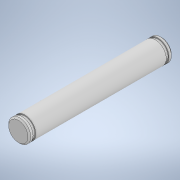
# Autodesk Inventor part: Aksel_stempel_bund
Saved by Autodesk Inventor 2022 (Build 260153000, 153)
## iProperties
Created: 2022-05-05
Part Number: Aksel_stempel_bund
Material: Generic
Document SubType Name: Modeling
Designer: patri
Density: 1 g/cm^3
Appearance: Default
Author: patri
Autodesk Inventor part; units mm, degrees
ref_plane "YZ Plane" through (0, 0, 0) normal (1, 0, 0) x (0, 1, 0)
ref_plane "XZ Plane" through (0, 0, 0) normal (0, 1, 0) x (-1, 0, 0)
ref_plane "XY Plane" through (0, 0, 0) normal (0, 0, 1) x (1, 0, 0)
sketch "Sketch1" plane through (0, 0, 0) normal (0, 1, 0) x (-1, 0, 0)
  line L0 (0, 0) -> (6, 0)
  line L1 (6, 0) -> (6, -78)
  line L2 (6, -78) -> (0, -78)
  line L3 (0, -78) -> (0, 0)
  line L4 (6, -2) -> (5.5, -2)
  line L5 (5.5, -2) -> (5.5, -3.5)
  line L6 (5.5, -3.5) -> (6, -3.5)
  line L7 (6, -3.5) -> (6, -2)
  line L8 (6, -76) -> (5.5, -76)
  line L9 (5.5, -76) -> (5.5, -74.5)
  line L10 (5.5, -74.5) -> (6, -74.5)
  line L11 (6, -74.5) -> (6, -76)
  point P0 (6, -74.5)
  point P1 (6, -3.5)
  dimension "d0" = 6
  dimension "d3" = 71
  dimension "d4" = 1.5
  dimension "d5" = 0.5
  dimension "d6" = 1.5
  dimension "d7" = 2
  dimension "d8" = 2
  constraints: 24 end point, 6 parallel, 3 horizontal, 3 perpendicular, 3 point on line
  measures "d0" distance between parallel lines of L3 L1
  measures "d3" distance between parallel lines of L6 L10
  measures "d4" distance of L4.end L5.end
  measures "d5" distance of L5.end L6.end
  measures "d6" distance of L8.end L9.end
  measures "d7" distance between parallel lines of L8 L2
  measures "d8" distance between parallel lines of L0 L4
revolve "Revolution1" add sketch "Sketch1" angle 360 about axis through (0, 0, -78) along (0, 0, 1) contours L0 L1 L4 L5 L6 L10 L9 L8 L2 L3
chamfer "Chamfer1" distance 0.75 angle 45 2 edges at (6, 0, 0) (6, 0, -78)
body "Solid1"
